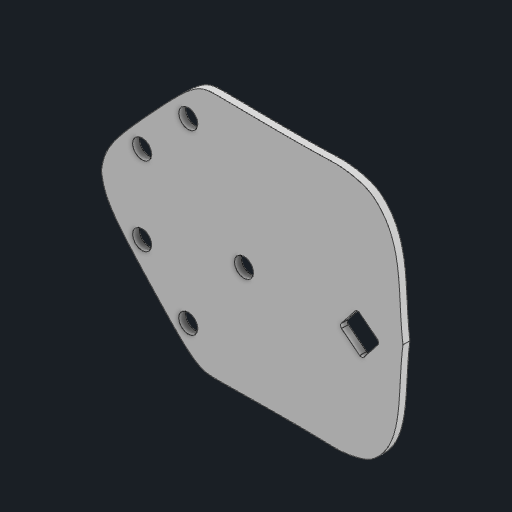
# Autodesk Inventor part: outer-tracking-wheel
Saved by Autodesk Inventor 2023.2 (Build 272271000, 271)
## iProperties
Created: 2023-03-27
Part Number: outer-tracking-wheel
Material: Generic
Document SubType Name: Modeling
Designer: Liam
Density: 1 g/cm^3
Appearance: Default
Author: Liam
Autodesk Inventor part; units mm, degrees
ref_plane "YZ Plane" through (0, 0, 0) normal (1, 0, 0) x (0, 1, 0)
ref_plane "XZ Plane" through (0, 0, 0) normal (0, 1, 0) x (-1, 0, 0)
ref_plane "XY Plane" through (0, 0, 0) normal (0, 0, 1) x (1, 0, 0)
sketch "Sketch1" plane through (0, 0, 0) normal (0, 0, 1) x (1, 0, 0)
  spline S0 degree 4 poles (-33.1249, 0) (-32.7441, -3.3083) (-31.301, -6.6794) (-25.1865, -13.1344) (-12.5879, -26.9519) (-9.3373, -27.1021) (-5.3044, -27.0484) (16.0931, -26.7836) (19.0099, -27.4332) (24.6336, -26.2422) (28.3291, -24.1322) (33.2798, -17.6852) (32.0106, -8.7104) (33.1249, 0) knots 0 0 0 0 0 0.186295 0.267444 0.346796 0.434615 0.512243 0.592107 0.668739 0.725194 0.784698 1 1 1 1 1
  spline S1 degree 4 poles (33.1249, 0) (32.0106, 8.7104) (33.2798, 17.6852) (28.3291, 24.1322) (24.6336, 26.2422) (19.0099, 27.4332) (16.0932, 26.7836) (-5.3044, 27.0484) (-9.3373, 27.1021) (-12.5879, 26.9519) (-25.1865, 13.1344) (-31.301, 6.6794) (-32.7441, 3.3083) (-33.1249, 0) knots 0 0 0 0 0 0.215302 0.274806 0.331261 0.407893 0.487757 0.565385 0.653204 0.732556 0.813705 1 1 1 1 1
  line L0 (27.5603, -1.7998) -> (23.5713, 1.3457)
  arc A0 (27.6658, -2.6916) -> (27.5603, -1.7998) centre (27.1671, -2.2984) ccw
  line L1 (24.5203, -6.6806) -> (27.6658, -2.6916)
  arc A1 (23.6285, -6.7861) -> (24.5203, -6.6806) centre (24.0217, -6.2875) ccw
  line L2 (19.6395, -3.6406) -> (23.6285, -6.7861)
  arc A2 (19.534, -2.7488) -> (19.6395, -3.6406) centre (20.0326, -3.142) ccw
  line L3 (22.6795, 1.2402) -> (19.534, -2.7488)
  arc A3 (23.5713, 1.3457) -> (22.6795, 1.2402) centre (23.1781, 0.8471) ccw
  circle A4 centre (-1.8001, -2.7202) radius 2.0955
  arc A5 (-26.7749, 2.0828) -> (-26.7749, -2.0828) centre (-26.7749, 0) ccw projected
  arc A6 (4.9751, -2.0828) -> (4.9751, 2.0828) centre (4.9751, 0) ccw projected
  line L4 (4.9751, 0) -> (-26.7749, 0)
  circle A7 centre (-14.0458, -19.4753) radius 2.0955
  circle A8 centre (-14.0458, 19.4753) radius 2.0955
  circle A9 centre (-24.1871, -8.628) radius 2.0955
  circle A10 centre (-24.1871, 8.628) radius 2.0955
  point P0 (-0.0456, -0.069)
  point P1 (-32.175, -3.7784)
  point P2 (-29.5173, -8.1033)
  point P3 (-21.489, -17.2087)
  point P4 (-12.0921, -26.1201)
  point P5 (-9.5119, -26.9934)
  point P6 (-5.4733, -27.0476)
  point P7 (15.9689, -27.0472)
  point P8 (20.8905, -26.9087)
  point P9 (24.5964, -26.005)
  point P10 (26.7618, -24.8125)
  point P11 (29.203, -22.1593)
  point P12 (31.7141, -15.7042)
  point P13 (31.7141, 15.7042)
  point P14 (29.203, 22.1593)
  point P15 (26.7618, 24.8125)
  point P16 (24.5964, 26.005)
  point P17 (20.8905, 26.9087)
  point P18 (15.9689, 27.0472)
  point P19 (-5.4733, 27.0476)
  point P20 (-9.512, 26.9934)
  point P21 (-12.0921, 26.1201)
  point P22 (-21.489, 17.2087)
  point P23 (-29.5173, 8.1033)
  point P24 (-32.175, 3.7784)
  dimension "d0" = 4.191
  dimension "d1" = 4.191
  dimension "d2" = 4.191
  dimension "d3" = 4.191
  dimension "d4" = 4.191
  constraints: 10 end point, 9 centre point, 8 point on circle, 2 symmetric about line, 1 horizontal, 66 other
  measures "d0" diameter of A4
  measures "d1" diameter of A7
  measures "d2" diameter of A8
  measures "d3" diameter of A9
  measures "d4" diameter of A10
extrude "Extrusion1" add sketch "Sketch1" along normal blind 1.524
equation "\"d2\" = d1"
equation "\"d3\" = d1"
equation "\"d4\" = d3"
body "Solid1"
